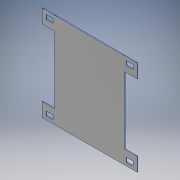
# Autodesk Inventor part: 밑판
Saved by Autodesk Inventor 2017 (Build 210142000, 142)
## iProperties
Part Number: 밑판
Material: 알루미늄 6061
Document SubType Name: Modeling
Designer: minom
Density: 2.7 g/cm^3
Appearance: 알루미늄 - 평지
Mass: 411.697 g
Surface Area: 1609.63 cm^2
Volume: 152.48 cm^3
Author: minom
Autodesk Inventor part; units mm, degrees
ref_plane "YZ Plane" through (0, 0, 0) normal (1, 0, 0) x (0, 1, 0)
ref_plane "XZ Plane" through (0, 0, 0) normal (0, 1, 0) x (-1, 0, 0)
ref_plane "XY Plane" through (0, 0, 0) normal (0, 0, 1) x (1, 0, 0)
sketch "스케치1" plane through (0, 0, 0) normal (0, 1, 0) x (-1, 0, 0)
  line L0 (0, 0) -> (-230, 0)
  line L1 (-230, 0) -> (-230, -309.2)
  line L2 (-230, -309.2) -> (0, -309.2)
  line L3 (0, -309.2) -> (0, 0)
  dimension "d0" = 230
  dimension "d1" = 309.2
  constraints: 8 end point, 2 parallel, 1 horizontal, 1 perpendicular
  measures "d0" distance of L2.end L1.end
  measures "d1" distance of L1.end L0.end
extrude "돌출1" add sketch "스케치1" along normal blind 2
sketch "스케치2" plane through (0, 2, 0) normal (0, 1, 0) x (1, 0, 0)
  line L0 (1, 0) -> (1, 309.2)
  line L1 (230, 309.2) -> (0, 309.2) projected
  line L2 (6.2, 309.2) -> (6.2, 0)
  line L3 (229, 0) -> (229, 309.2)
  line L4 (223.8, 309.2) -> (223.8, 0)
  line L5 (0, 0) -> (230, 0) projected
  line L6 (0, 309.2) -> (0, 0) projected
  line L7 (230, 0) -> (230, 309.2) projected
  line L8 (1, 0) -> (6.2, 0)
  line L9 (1, 309.2) -> (6.2, 309.2)
  line L10 (223.8, 309.2) -> (229, 309.2)
  line L11 (223.8, 0) -> (229, 0)
  dimension "d4" = 1
  dimension "d5" = 5.2
  dimension "d6" = 1
  dimension "d7" = 5.2
  constraints: 16 end point, 5 point on line, 4 collinear, 2 vertical, 1 parallel, 1 perpendicular
  measures "d4" distance between parallel lines of L0 L6
  measures "d5" distance between parallel lines of L2 L0
  measures "d6" distance between parallel lines of L7 L3
  measures "d7" distance between parallel lines of L4 L3
extrude "돌출2" cut sketch "스케치2" against normal blind 1 contours L0 L1 L2 L5 | L4 L1 L3 L5
sketch "스케치3" plane through (0, 0, 0) normal (0, -1, 0) x (1, 0, 0)
  line L0 (0, 0) -> (0, -45)
  line L1 (0, -309.2) -> (0, 0) projected
  line L2 (0, -45) -> (-40, -45)
  line L3 (-40, -45) -> (-40, 0)
  line L4 (-40, 0) -> (0, 0)
  line L5 (230, 0) -> (230, -309.2) projected
  line L6 (230, 0) -> (230, -45)
  line L7 (230, -45) -> (270, -45)
  line L8 (270, -45) -> (270, 0)
  line L9 (270, 0) -> (230, 0)
  line L10 (230, -309.2) -> (270, -309.2)
  line L11 (270, -309.2) -> (270, -264.2)
  line L12 (270, -264.2) -> (230, -264.2)
  line L13 (0, -309.2) -> (-40, -309.2)
  line L14 (-40, -309.2) -> (-40, -264.2)
  line L15 (-40, -264.2) -> (0, -264.2)
  dimension "d10" = 45
  constraints: 28 end point, 14 point on line, 5 perpendicular, 1 horizontal, 1 parallel
  measures "d10" distance of L10.end L11.end
extrude "돌출3" add sketch "스케치3" against normal blind 2
sketch "스케치4" plane through (0, 2, 0) normal (0, 1, 0) x (1, 0, 0)
  line L0 (1, 0) -> (1, 309.2) projected
  line L1 (1, 309.2) -> (-40, 309.2) projected
  line L2 (-40, 309.2) -> (-40, 264.2) projected
  line L3 (-40, 264.2) -> (0, 264.2) projected
  line L4 (0, 264.2) -> (0, 45) projected
  line L5 (0, 45) -> (-40, 45) projected
  line L6 (-40, 45) -> (-40, 0) projected
  line L7 (-40, 0) -> (1, 0) projected
  line L8 (223.8, 0) -> (223.8, 309.2) projected
  line L9 (223.8, 309.2) -> (6.2, 309.2) projected
  line L10 (6.2, 309.2) -> (6.2, 0) projected
  line L11 (6.2, 0) -> (223.8, 0) projected
  line L12 (229, 309.2) -> (229, 0) projected
  line L13 (229, 0) -> (270, 0) projected
  line L14 (270, 0) -> (270, 45) projected
  line L15 (270, 45) -> (230, 45) projected
  line L16 (230, 45) -> (230, 264.2) projected
  line L17 (230, 264.2) -> (270, 264.2) projected
  line L18 (270, 264.2) -> (270, 309.2) projected
  line L19 (270, 309.2) -> (229, 309.2) projected
  line L20 (-39, 0) -> (-39, 45)
  line L21 (0, 45) -> (-40, 45) projected
  line L22 (-33.8, 45) -> (-33.8, 0)
  line L23 (-39, 264.2) -> (-39, 309.2)
  line L24 (1, 309.2) -> (-40, 309.2) projected
  line L25 (-33.8, 309.2) -> (-33.8, 264.2)
  line L26 (0, 264.2) -> (-40, 264.2) projected
  line L27 (229, 0) -> (270, 0) projected
  line L28 (269, 0) -> (269, 45)
  line L29 (230, 45) -> (270, 45) projected
  line L30 (263.8, 0) -> (263.8, 45)
  line L31 (230, 264.2) -> (270, 264.2) projected
  line L32 (269, 264.2) -> (269, 309.2)
  line L33 (270, 309.2) -> (229, 309.2) projected
  line L34 (263.8, 309.2) -> (263.8, 264.2)
  line L35 (263.8, 264.2) -> (269, 264.2)
  line L36 (269, 309.2) -> (263.8, 309.2)
  point P0 (0, 0)
  dimension "d13" = 1
  dimension "d14" = 5.2
  dimension "d15" = 1
  dimension "d16" = 1
  dimension "d17" = 5.2
  constraints: 20 end point, 18 point on line, 4 perpendicular, 2 collinear, 2 parallel, 1 vertical
  measures "d13" distance between parallel lines of L20 L6
  measures "d14" distance between parallel lines of L22 L20
  measures "d15" distance between parallel lines of L23 L2
  measures "d16" distance between parallel lines of L14 L28
  measures "d17" distance between parallel lines of L28 L30
extrude "돌출4" cut sketch "스케치4" against normal blind 1 contours L7 L20 L5 L22 | L25 L3 L23 L1 | L19 L32 L17 L34 | L30 L15 L28 L13
sketch "스케치5" plane through (0, 2, 0) normal (0, 1, 0) x (1, 0, 0)
  line L0 (223.8, 0) -> (223.8, 309.2) projected
  line L1 (223.8, 309.2) -> (6.2, 309.2) projected
  line L2 (6.2, 309.2) -> (6.2, 0) projected
  line L3 (6.2, 0) -> (223.8, 0) projected
  line L4 (-33.8, 309.2) -> (-33.8, 264.2) projected
  line L5 (-33.8, 264.2) -> (0, 264.2) projected
  line L6 (0, 264.2) -> (0, 45) projected
  line L7 (0, 45) -> (-33.8, 45) projected
  line L8 (-33.8, 45) -> (-33.8, 0) projected
  line L9 (-33.8, 0) -> (1, 0) projected
  line L10 (1, 0) -> (1, 309.2) projected
  line L11 (1, 309.2) -> (-33.8, 309.2) projected
  line L12 (263.8, 0) -> (263.8, 45) projected
  line L13 (263.8, 45) -> (230, 45) projected
  line L14 (230, 45) -> (230, 264.2) projected
  line L15 (230, 264.2) -> (263.8, 264.2) projected
  line L16 (263.8, 264.2) -> (263.8, 309.2) projected
  line L17 (263.8, 309.2) -> (229, 309.2) projected
  line L18 (229, 309.2) -> (229, 0) projected
  line L19 (229, 0) -> (263.8, 0) projected
  line L20 (-33.8, 45) -> (-33.8, 0) projected
  line L21 (-40, 45) -> (0, 45) projected
  line L22 (-4.8, 24) -> (-4.8, 12)
  line L23 (-5.8, 11) -> (-25.8, 11)
  line L24 (-26.8, 12) -> (-26.8, 24)
  line L25 (-5.8, 25) -> (-25.8, 25)
  line L26 (230, 45) -> (270, 45) projected
  line L27 (255.8, 25) -> (235.8, 25)
  line L28 (234.8, 24) -> (234.8, 12)
  line L29 (235.8, 11) -> (255.8, 11)
  line L30 (256.8, 12) -> (256.8, 24)
  line L31 (230, 264.2) -> (263.8, 264.2) projected
  line L32 (255.8, 284.2) -> (235.8, 284.2)
  line L33 (234.8, 285.2) -> (234.8, 297.2)
  line L34 (235.8, 298.2) -> (255.8, 298.2)
  line L35 (256.8, 297.2) -> (256.8, 285.2)
  line L36 (-33.8, 264.2) -> (0, 264.2) projected
  arc A0 (235.8, 298.2) -> (234.8, 297.2) centre (235.8, 297.2) ccw
  arc A1 (256.8, 297.2) -> (255.8, 298.2) centre (255.8, 297.2) ccw
  arc A2 (255.8, 284.2) -> (256.8, 285.2) centre (255.8, 285.2) ccw
  arc A3 (234.8, 285.2) -> (235.8, 284.2) centre (235.8, 285.2) ccw
  arc A4 (235.8, 25) -> (234.8, 24) centre (235.8, 24) ccw
  arc A5 (234.8, 12) -> (235.8, 11) centre (235.8, 12) ccw
  arc A6 (255.8, 11) -> (256.8, 12) centre (255.8, 12) ccw
  arc A7 (256.8, 24) -> (255.8, 25) centre (255.8, 24) ccw
  arc A8 (-25.8, 25) -> (-26.8, 24) centre (-25.8, 24) ccw
  arc A9 (-26.8, 12) -> (-25.8, 11) centre (-25.8, 12) ccw
  arc A10 (-5.8, 11) -> (-4.8, 12) centre (-5.8, 12) ccw
  arc A11 (-4.8, 24) -> (-5.8, 25) centre (-5.8, 24) ccw
  line L37 (1, 309.2) -> (-33.8, 309.2) projected
  line L38 (-33.8, 309.2) -> (-26.8, 309.2)
  line L39 (-26.8, 309.2) -> (-26.8, 298.2)
  line L40 (-25.8, 298.2) -> (-5.8, 298.2)
  line L41 (-4.8, 297.2) -> (-4.8, 285.2)
  line L42 (-5.8, 284.2) -> (-25.8, 284.2)
  line L43 (-26.8, 285.2) -> (-26.8, 297.2)
  arc A12 (-5.8, 284.2) -> (-4.8, 285.2) centre (-5.8, 285.2) ccw
  arc A13 (-4.8, 297.2) -> (-5.8, 298.2) centre (-5.8, 297.2) ccw
  arc A14 (-25.8, 298.2) -> (-26.8, 297.2) centre (-25.8, 297.2) ccw
  arc A15 (-26.8, 285.2) -> (-25.8, 284.2) centre (-25.8, 285.2) ccw
  point P0 (0, 0)
  point P1 (-4.8, 11)
  point P2 (234.8, 25)
  point P3 (234.8, 11)
  point P4 (256.8, 11)
  point P5 (234.8, 284.2)
  point P6 (234.8, 298.2)
  point P7 (256.8, 298.2)
  point P8 (-4.8, 284.2)
  point P9 (-4.8, 298.2)
  point P10 (-26.8, 284.2)
  dimension "d27" = 14
  dimension "d29" = 14
  dimension "d33" = 11
  dimension "d34" = 11
  dimension "d35" = 11
  dimension "d37" = 7
  dimension "d38" = 11
  dimension "d39" = 22
  dimension "d40" = 14
  dimension "d41" = 1
  dimension "d42" = 14
  constraints: 36 end point, 32 point on circle, 32 tangent, 25 point on line, 16 centre point, 10 perpendicular, 6 equal radius, 2 parallel, 1 horizontal
  measures "d27" distance of point (234.8, 25) point (234.8, 11)
  measures "d29" distance of point (234.8, 284.2) point (234.8, 298.2)
  measures "d33" distance between parallel lines of L29 L19
  measures "d34" distance between parallel lines of L23 L9
  measures "d35" distance between parallel lines of L17 L34
  measures "d37" distance of L4.start L38.end
  measures "d38" distance of L38.end L39.end
  measures "d39" distance of point (-4.8, 284.2) point (-26.8, 284.2)
  measures "d40" distance of point (-4.8, 298.2) point (-4.8, 284.2)
  measures "d41" radius of A12
  measures "d42" distance between parallel lines of L25 L23
extrude "돌출6" cut sketch "스케치5" against normal blind 10 contours L22 A10 L23 A9 L24 A8 L25 A11 | A7 L30 A6 L29 A5 L28 A4 L27 | L32 A3 L33 A0 L34 A1 L35 A2 | L40 A13 L41 A12 L42 A15 L43 A14
